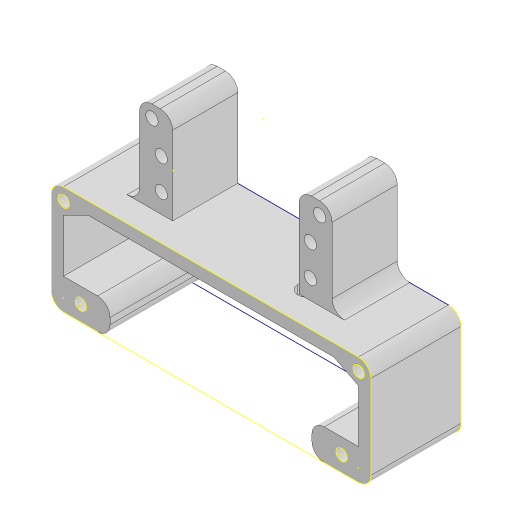
# Autodesk Inventor part: 4BarCameraHolder
Saved by Autodesk Inventor 2023 (Build 270158000, 158)
## iProperties
Created: 2022-10-07
Part Number: 4BarCameraHolder
Material: Generic
Document SubType Name: Modeling
Designer: deli
Density: 1 g/cm^3
Appearance: Default
Author: deli
Autodesk Inventor part; units mm, degrees
ref_plane "YZ Plane" through (0, 0, 0) normal (1, 0, 0) x (0, 1, 0)
ref_plane "XZ Plane" through (0, 0, 0) normal (0, 1, 0) x (-1, 0, 0)
ref_plane "XY Plane" through (0, 0, 0) normal (0, 0, 1) x (1, 0, 0)
sketch "Sketch1" plane through (0, 0, 0) normal (0, 1, 0) x (-1, 0, 0)
  line L0 (-59.6946, 47.1235) -> (-59.6946, 26.1235)
  line L1 (35.3054, 26.1235) -> (35.3054, 47.1235)
  line L2 (20.3054, 57.1235) -> (20.3054, 47.1235)
  line L3 (20.3054, 47.1235) -> (35.3054, 47.1235)
  line L4 (-44.6946, 57.1235) -> (-44.6946, 47.1235)
  line L5 (-44.6946, 47.1235) -> (-59.6946, 47.1235)
  line L6 (-63.6946, 57.1235) -> (-63.6946, 22.1235)
  line L7 (39.3054, 22.1235) -> (39.3054, 57.1235)
  line L8 (39.3054, 57.1235) -> (20.3054, 57.1235)
  line L9 (-44.6946, 57.1235) -> (-63.6946, 57.1235)
  line L10 (-29.6946, 26.1235) -> (-29.6946, 22.1235)
  line L11 (-35.6946, 26.1235) -> (-35.6946, 22.1235)
  line L12 (-59.6946, 26.1235) -> (-35.6946, 26.1235)
  line L13 (-29.6946, 26.1235) -> (35.3054, 26.1235)
  line L14 (-63.6946, 22.1235) -> (-35.6946, 22.1235)
  line L15 (-29.6946, 22.1235) -> (39.3054, 22.1235)
  point P0 (0, 0)
  dimension "d0" = 95
  dimension "d2" = 15
  dimension "d4" = 15
  dimension "d8" = 4
  dimension "d10" = 4
  dimension "d11" = 10
  dimension "d12" = 10
  dimension "d13" = 6
  dimension "d14" = 28
  dimension "d33" = 21
  dimension "d34" = 0
  dimension "d35" = 4
  dimension "d36" = 4
  dimension "d37" = 21
  constraints: 32 end point, 7 parallel, 4 perpendicular, 2 horizontal
  measures "d0" distance of L1.start L0.end
  measures "d2" distance of L1.end L2.end
  measures "d4" distance of L0.start L4.end
  measures "d8" distance between parallel lines of L1 L7
  measures "d10" distance between parallel lines of L0 L6
  measures "d11" distance between parallel lines of L5 L9
  measures "d12" distance between parallel lines of L3 L8
  measures "d13" distance between parallel lines of L11 L10
  measures "d14" distance between parallel lines of L11 L6
  measures "d33" distance of L1.start L1.end
  measures "d34" distance between parallel lines of L14 L15
  measures "d35" distance between parallel lines of L15 L13
  measures "d36" distance between parallel lines of L14 L12
  measures "d37" distance between parallel lines of L12 L5
extrude "Extrusion1" add sketch "Sketch1" along normal blind 29
sketch "Sketch6" plane through (0, 29, 0) normal (0, 1, 0) x (1, 0, 0)
  line L0 (29.6946, -22.1235) -> (-39.3054, -22.1235) projected
  line L1 (35.6946, -26.1235) -> (59.6946, -26.1235) projected
  line L2 (29.6946, -22.1235) -> (35.6946, -22.1235)
  line L3 (35.6946, -22.1235) -> (35.6946, -26.1235)
  line L4 (35.6946, -26.1235) -> (29.6946, -26.1235)
  line L5 (29.6946, -26.1235) -> (29.6946, -22.1235)
  point P0 (0, 0)
  constraints: 8 end point, 2 parallel, 1 horizontal, 1 perpendicular
extrude "Extrusion6" add sketch "Sketch6" against normal blind 7.5
fillet "Fillet5" radius 3 2 edges at (29.6946, 21.5, 24.1235) (35.6946, 21.5, 24.1235)
sketch "Sketch7" plane through (29.6946, 0, 22.1235) normal (0, 0, -1) x (-1, 0, 0)
  line L0 (48.5, 0) -> (37.85, 0)
  line L1 (37.85, 0) -> (37.85, 21)
  line L2 (37.85, 21) -> (48.5, 21)
  line L3 (48.5, 21) -> (48.5, 0)
  line L4 (-13.5, 0) -> (-2.85, 0)
  line L5 (-2.85, 0) -> (-2.85, 21)
  line L6 (-2.85, 21) -> (-13.5, 21)
  line L7 (-13.5, 21) -> (-13.5, 0)
  line L8 (69, 0) -> (69, 29) projected
  line L9 (-34, 0) -> (-34, 29) projected
  line L10 (-34, 29) -> (69, 29) projected
  line L11 (0, 0) -> (69, 0) projected
  point P0 (29.6946, 0)
  dimension "d58" = 10.65
  dimension "d60" = 40.7
  dimension "d61" = 20.5
  dimension "d62" = 103
  dimension "d63" = 8
  constraints: 16 end point, 4 parallel, 2 collinear, 2 equal length, 2 horizontal, 2 perpendicular
  measures "d58" distance of L0.start L0.end
  measures "d60" distance between parallel lines of L1 L5
  measures "d61" distance between parallel lines of L8 L3
  measures "d62" distance between parallel lines of L9 L8
  measures "d63" distance between parallel lines of L10 L2
extrude "Extrusion7" add sketch "Sketch7" along normal blind 29.3
sketch "Sketch8" plane through (-18.8054, 21, -7.1765) normal (0, 1, 0) x (1, 0, 0)
  circle A0 centre (4, -4) radius 2
  circle A1 centre (58, -4) radius 2
  line L0 (10.65, -29.3) -> (10.65, 0) projected
  line L1 (0, -29.3) -> (0, 0) projected
  line L2 (62, -29.3) -> (62, 0) projected
  line L3 (0, 0) -> (10.65, 0) projected
  line L4 (51.35, 0) -> (62, 0) projected
  circle A2 centre (7, -13.05) radius 2
  circle A3 centre (7, -23.05) radius 2
  circle A4 centre (55, -13.05) radius 2
  circle A5 centre (55, -23.05) radius 2
  line L5 (51.35, -29.3) -> (51.35, 0) projected
  point P0 (18.8054, -7.1765)
  point P1 (0, -23.3)
  point P2 (62, -23.3)
  point P3 (56.675, 0)
  dimension "d68" = 4
  dimension "d69" = 4
  dimension "d70" = 4
  dimension "d71" = 4
  dimension "d75" = 9.05
  dimension "d76" = 3.65
  dimension "d77" = 10
  dimension "d78" = 3.65
  dimension "d79" = 10
  dimension "d80" = 9.05
  dimension "d81" = 3.65
  dimension "d82" = 3.65
  dimension "d83" = 4
  constraints: 6 centre point, 5 equal radius, 1 midpoint
  measures "d68" distance from line of L1 A0.centre
  measures "d69" distance from line of L2 A1.centre
  measures "d70" distance from line of L3 A0.centre
  measures "d71" vertical distance of point (56.675, 0) A1.centre
  measures "d75" vertical distance of A0.centre A2.centre
  measures "d76" distance from line of L0 A2.centre
  measures "d77" distance of A2.centre A3.centre
  measures "d78" distance from line of L0 A3.centre
  measures "d79" distance of A5.centre A4.centre
  measures "d80" vertical distance of A4.centre A1.centre
  measures "d81" distance from line of A4.centre L5
  measures "d82" distance from line of A5.centre L5
  measures "d83" diameter of A0
extrude "Extrusion8" cut sketch "Sketch8" against normal blind 29.3
fillet "Fillet7" radius 4 14 edges at (-18.8054, 10.5, -7.1765) (-8.1554, 10.5, -7.1765) (32.5446, 10.5, -7.1765) (43.1946, 10.5, -7.1765) (63.6946, 14.5, 22.1235) (63.6946, 14.5, 57.1235) (-39.3054, 14.5, 57.1235) (-20.3054, 14.5, 57.1235) (-39.3054, 14.5, 22.1235) (44.6946, 14.5, 57.1235) (-20.3054, 14.5, 47.1235) (44.6946, 14.5, 47.1235) (43.1946, 10.5, 22.1235) (-18.8054, 10.5, 22.1235)
sketch "Sketch10" plane through (0, 29, 0) normal (0, 1, 0) x (1, 0, 0)
  circle A0 centre (-29.8054, -52.1235) radius 1.85
  circle A1 centre (54.1946, -52.1235) radius 1.85
  circle A2 centre (59.6946, -26.1235) radius 1.85
  circle A3 centre (-35.3054, -26.1235) radius 1.85
  arc A4 (-39.3054, -53.1235) -> (-35.3054, -57.1235) centre (-35.3054, -53.1235) ccw construction
  arc A5 (-20.3054, -51.1235) -> (-24.3054, -47.1235) centre (-24.3054, -51.1235) ccw construction
  arc A6 (48.6946, -47.1235) -> (44.6946, -51.1235) centre (48.6946, -51.1235) ccw construction
  arc A7 (59.6946, -57.1235) -> (63.6946, -53.1235) centre (59.6946, -53.1235) ccw construction
  line L0 (-35.3054, -53.1235) -> (-24.3054, -51.1235) construction
  line L1 (48.6946, -51.1235) -> (59.6946, -53.1235) construction
  arc A8 (-35.3054, -22.1235) -> (-39.3054, -26.1235) centre (-35.3054, -26.1235) ccw construction
  arc A9 (63.6946, -26.1235) -> (59.6946, -22.1235) centre (59.6946, -26.1235) ccw construction
  point P0 (0, 0)
  dimension "d86" = 3.7
  constraints: 4 centre point, 4 end point, 3 equal radius, 2 coincident, 2 concentric, 2 midpoint
  measures "d86" diameter of A3
chamfer "Chamfer1" distance 4 distance2 8 1 edges at (-35.3054, 14.5, 26.1235) measured on face at (-35.3054, 14.5, 26.6235)
chamfer "Chamfer2" distance 4 distance2 8 1 edges at (59.6946, 14.5, 26.1235) measured on face at (59.6946, 14.5, 26.6235)
extrude "Extrusion10" cut sketch "Sketch10" against normal blind 30
sketch "Sketch11" plane through (0, 0, 0) normal (0, -1, 0) x (1, 0, 0)
  circle A0 centre (59.6946, 26.1235) radius 1.85 projected
  circle A1 centre (54.1946, 52.1235) radius 1.85 projected
  circle A2 centre (-29.8054, 52.1235) radius 1.85 projected
  circle A3 centre (-35.3054, 26.1235) radius 1.85 projected
  arc A4 (-39.3054, 26.1235) -> (-35.3054, 22.1235) centre (-35.3054, 26.1235) ccw projected
  line L0 (-39.3054, 26.1235) -> (-39.3054, 53.1235) projected
  arc A5 (-35.3054, 57.1235) -> (-39.3054, 53.1235) centre (-35.3054, 53.1235) ccw projected
  arc A6 (59.6946, 22.1235) -> (63.6946, 26.1235) centre (59.6946, 26.1235) ccw projected
  line L1 (63.6946, 53.1235) -> (63.6946, 26.1235) projected
  arc A7 (63.6946, 53.1235) -> (59.6946, 57.1235) centre (59.6946, 53.1235) ccw projected
  line L2 (35.6946, 22.1235) -> (35.6946, 26.1235) projected
  line L3 (35.6946, 26.1235) -> (29.6946, 26.1235) projected
  line L4 (29.6946, 26.1235) -> (29.6946, 22.1235) projected
  line L5 (35.6946, 22.1235) -> (32.5446, 22.1235) construction
  line L6 (59.6946, 22.1235) -> (35.6946, 22.1235)
  line L7 (29.6946, 22.1235) -> (-35.3054, 22.1235)
  line L8 (59.6946, 57.1235) -> (-35.3054, 57.1235)
  point P0 (0, 0)
  constraints: 6 end point, 2 horizontal
sketch "Sketch12" plane through (0, 29, 0) normal (0, 1, 0) x (1, 0, 0)
  circle A0 centre (-29.8054, -52.1235) radius 1.85 projected
  circle A1 centre (-35.3054, -26.1235) radius 1.85 projected
  circle A2 centre (59.6946, -26.1235) radius 1.85 projected
  circle A3 centre (54.1946, -52.1235) radius 1.85 projected
  line L0 (63.6946, -53.1235) -> (63.6946, -26.1235) projected
  arc A4 (59.6946, -57.1235) -> (63.6946, -53.1235) centre (59.6946, -53.1235) ccw projected
  arc A5 (63.6946, -26.1235) -> (59.6946, -22.1235) centre (59.6946, -26.1235) ccw projected
  line L1 (59.6946, -22.1235) -> (-35.3054, -22.1235) projected
  arc A6 (-35.3054, -22.1235) -> (-39.3054, -26.1235) centre (-35.3054, -26.1235) ccw projected
  line L2 (-39.3054, -26.1235) -> (-39.3054, -53.1235) projected
  arc A7 (-39.3054, -53.1235) -> (-35.3054, -57.1235) centre (-35.3054, -53.1235) ccw projected
  line L3 (59.6946, -57.1235) -> (-35.3054, -57.1235) projected
  point P0 (0, 0)
equation "\"d4\" = d2"
equation "\"d10\" = d8"
equation "\"d12\" = d11"
equation "\"d36\" = d35"
equation "\"d37\" = d33"
equation "\"d61\" = -d58 + 0.5 * d62 - 0.5 * d60"
equation "\"d70\" = d68"
equation "\"d71\" = d70"
equation "\"d78\" = d76"
equation "\"d79\" = d77"
equation "\"d80\" = d75"
equation "\"d81\" = d76"
equation "\"d82\" = d78"
equation "\"d9\" = d8"
equation "\"d40\" = d38"
equation "\"d43\" = d40"
equation "\"d38\" = 8"
body "Solid1"
